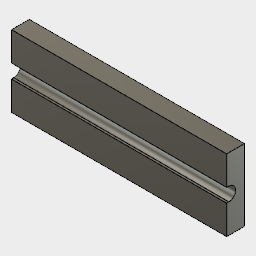
Tentacle_mold_01 v1 (Autodesk Fusion 360 design; units mm, degrees)
Autodesk Fusion 360 part; units mm, degrees
sketch "Sketch1" plane through (0, 0, 0) normal (1, 0, 0) x (0, 0, -1)
sketch "Sketch2" plane through (0, 0, 0) normal (1, 0, 0) x (0, 0, -1)
sketch "Sketch3" plane through (0, 0, 0) normal (1, 0, 0) x (0, 0, -1)
  line L0 (0, 0) -> (-25, 0)
  line L1 (-25, 100) -> (0, 100)
  line L2 (0, 100) -> (0, 0)
  line L3 (-25, 50) -> (0, 50) construction
  line L4 (-21.9677, 59.5249) -> (-25, 59.5352)
  line L5 (-21.9677, 40.4751) -> (-25, 40.4648)
  arc A0 (-21.9677, 40.4751) -> (-21.9677, 59.5249) centre (-22, 50) ccw
  line L6 (-25, 0) -> (-25, 40.4648)
  line L7 (-25, 59.5352) -> (-25, 100)
  dimension "d1" = 25
  dimension "d2" = 100
  dimension "d3" = 3
  dimension "d4" = 19.05
  measures "d1" distance of L1.start L1.end
  measures "d2" distance of L0.end L1.start
  measures "d3" distance of L3.start A0.centre
  measures "d4" diameter of A0
extrude "Extrude1" add sketch "Sketch3" along normal blind 300
equation "d4 = ( 3 / 4 * 25.4 ) * 1 mm"
